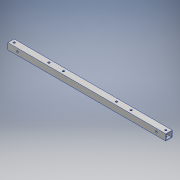
# Autodesk Inventor part: fsparts
Saved by Autodesk Inventor 2018 (Build 220112000, 112)
## iProperties
Created: 2019-04-22
Part Number: fsparts
Material: アルミニウム 6061
Document SubType Name: Modeling
Designer: Eiji Nishizawa
Density: 2.7 g/cm^3
Appearance: アルミニウム - フラット
Author: Eiji Nishizawa
Autodesk Inventor part; units mm, degrees
ref_plane "YZ Plane" through (0, 0, 0) normal (1, 0, 0) x (0, 1, 0)
ref_plane "XZ Plane" through (0, 0, 0) normal (0, 1, 0) x (-1, 0, 0)
ref_plane "XY Plane" through (0, 0, 0) normal (0, 0, 1) x (1, 0, 0)
sketch "スケッチ1" plane through (0, 0, 0) normal (1, 0, 0) x (0, 1, 0)
  line L0 (5, 5) -> (-5, 5)
  line L1 (-5, 5) -> (-5, -5)
  line L2 (-5, -5) -> (5, -5)
  line L3 (5, -5) -> (5, 5)
  line L4 (4, 4) -> (-4, 4)
  line L5 (-4, 4) -> (-4, -4)
  line L6 (-4, -4) -> (4, -4)
  line L7 (4, -4) -> (4, 4)
  point P0 (0, 0)
  dimension "d0" = 1
  dimension "d1" = 1
  dimension "d2" = 1
  dimension "d3" = 1
  dimension "d4" = 10
  dimension "d5" = 10
  dimension "d6" = 5
  dimension "d7" = 5
  constraints: 16 end point, 4 parallel, 2 horizontal, 2 perpendicular
  measures "d0" distance between parallel lines of L3 L7
  measures "d1" distance between parallel lines of L1 L5
  measures "d2" distance between parallel lines of L0 L4
  measures "d3" distance between parallel lines of L2 L6
  measures "d4" distance between parallel lines of L2 L0
  measures "d5" distance of L0.start L0.end
  measures "d6" distance from line of point (0, 0) L3
  measures "d7" distance from line of point (0, 0) L0
extrude "押し出し1" add sketch "スケッチ1" along normal blind 250
sketch "スケッチ2" plane through (0, -5, 5) normal (0, 0, 1) x (1, 0, 0)
  circle A0 centre (60, 5) radius 1.5
  circle A1 centre (190, 5) radius 1.5
  line L0 (250, 10) -> (250, 0) projected
  line L1 (0, 10) -> (0, 0) projected
  line L2 (0, 0) -> (250, 0) projected
  point P0 (0, 5)
  dimension "d10" = 60
  dimension "d11" = 3
  dimension "d12" = 3
  dimension "d13" = 60
  dimension "d14" = 5
  constraints: 2 centre point
  measures "d10" distance from line of L0 A1.centre
  measures "d11" diameter of A1
  measures "d12" diameter of A0
  measures "d13" distance from line of L1 A0.centre
  measures "d14" distance from line of L2 A0.centre
extrude "押し出し2" cut sketch "スケッチ2" against normal blind 200
sketch "スケッチ3" plane through (0, -5, 5) normal (0, 0, 1) x (1, 0, 0)
  circle A0 centre (5, 5) radius 1.5
  circle A1 centre (245, 5) radius 1.5
  line L0 (250, 10) -> (250, 0) projected
  line L1 (0, 10) -> (250, 10) projected
  line L2 (0, 10) -> (0, 0) projected
  point P0 (0, 5)
  dimension "d17" = 5
  dimension "d18" = 5
  dimension "d19" = 3
  dimension "d20" = 5
  dimension "d21" = 5
  dimension "d22" = 3
  constraints: 2 centre point
  measures "d17" distance from line of L0 A1.centre
  measures "d18" distance from line of L1 A1.centre
  measures "d19" diameter of A1
  measures "d20" distance from line of L2 A0.centre
  measures "d21" distance from line of L1 A0.centre
  measures "d22" diameter of A0
extrude "押し出し3" cut sketch "スケッチ3" against normal blind 200
sketch "スケッチ4" plane through (0, -5, 5) normal (0, 0, 1) x (1, 0, 0)
  circle A0 centre (83, 5) radius 1.5
  circle A1 centre (60, 5) radius 1.5 projected
  circle A2 centre (167, 5) radius 1.5
  circle A3 centre (190, 5) radius 1.5 projected
  line L0 (0, 0) -> (250, 0) projected
  point P0 (0, 5)
  dimension "d25" = 3
  dimension "d27" = 3
  dimension "d39" = 84
  dimension "d40" = 23
  dimension "d41" = 5
  dimension "d42" = 5
  dimension "d43" = 23
  constraints: 2 centre point
  measures "d25" diameter of A0
  measures "d27" diameter of A2
  measures "d39" distance of A2.centre A0.centre
  measures "d40" distance of A3.centre A2.centre
  measures "d41" distance from line of L0 A2.centre
  measures "d42" distance from line of A0.centre L0
  measures "d43" distance of A0.centre A1.centre
extrude "押し出し4" cut sketch "スケッチ4" against normal blind 200 contours A0 | A2
sketch "スケッチ5" plane through (0, 5, 5) normal (0, 1, 0) x (1, 0, 0)
  circle A0 centre (15, 5) radius 1.5
  line L0 (0, 10) -> (250, 10) projected
  line L1 (0, 10) -> (0, 0) projected
  circle A1 centre (235, 5) radius 1.5
  line L2 (250, 10) -> (250, 0) projected
  line L3 (0, 0) -> (250, 0) projected
  point P0 (0, 5)
  dimension "d31" = 3
  dimension "d32" = 5
  dimension "d33" = 15
  dimension "d34" = 15
  dimension "d35" = 5
  dimension "d36" = 3
  constraints: 2 centre point
  measures "d31" diameter of A0
  measures "d32" distance from line of L0 A0.centre
  measures "d33" distance from line of L1 A0.centre
  measures "d34" distance from line of L2 A1.centre
  measures "d35" distance from line of L3 A1.centre
  measures "d36" diameter of A1
extrude "押し出し5" cut sketch "スケッチ5" against normal blind 200 contours A0 | A1
